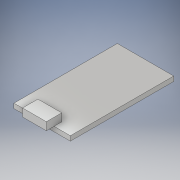
# Autodesk Inventor part: microplaceholder
Saved by Autodesk Inventor 2019 (Build 230136000, 136)
## iProperties
Created: 2020-06-11
Part Number: microplaceholder
Material: Aluminum 6061
Document SubType Name: Modeling
Designer: assman
Density: 2.7 g/cm^3
Appearance: Aluminum - Polished
Author: assman
Autodesk Inventor part; units mm, degrees
ref_plane "YZ Plane" through (0, 0, 0) normal (1, 0, 0) x (0, 1, 0)
ref_plane "XZ Plane" through (0, 0, 0) normal (0, 1, 0) x (-1, 0, 0)
ref_plane "XY Plane" through (0, 0, 0) normal (0, 0, 1) x (1, 0, 0)
sketch "Sketch1" plane through (0, 0, 0) normal (0, 1, 0) x (-1, 0, 0)
  line L0 (9, 16.5) -> (-9, 16.5)
  line L1 (-9, 16.5) -> (-9, -16.5)
  line L2 (-9, -16.5) -> (9, -16.5)
  line L3 (9, -16.5) -> (9, 16.5)
  line L4 (9, 16.5) -> (-9, -16.5) construction
  line L5 (-9, 16.5) -> (9, -16.5) construction
  point P0 (0, 0)
  dimension "d0" = 18
  dimension "d1" = 33
  constraints: 12 end point, 2 midpoint, 2 parallel, 1 horizontal, 1 perpendicular
  measures "d0" distance of L2.end L1.end
  measures "d1" distance of L1.end L0.end
extrude "Extrusion1" add sketch "Sketch1" along normal blind 1.5
sketch "Sketch2" plane through (0, 1.5, 0) normal (0, 1, 0) x (1, 0, 0)
  line L0 (-3.8, -18.95) -> (3.8, -18.95)
  line L1 (3.8, -18.95) -> (3.8, -14.05)
  line L2 (3.8, -14.05) -> (-3.8, -14.05)
  line L3 (-3.8, -14.05) -> (-3.8, -18.95)
  line L4 (-9, -16.5) -> (9, -16.5) projected
  line L5 (-3.8, -18.95) -> (3.8, -14.05) construction
  line L6 (3.8, -18.95) -> (-3.8, -14.05) construction
  point P0 (0, 0)
  point P1 (0, -16.5)
  dimension "d4" = 7.6
  dimension "d5" = 4.9
  constraints: 12 end point, 3 midpoint, 2 parallel, 1 horizontal, 1 perpendicular
  measures "d4" distance of L2.end L1.end
  measures "d5" distance of L1.end L0.end
extrude "Extrusion2" add sketch "Sketch2" along normal blind 2.5
body "Solid1"
